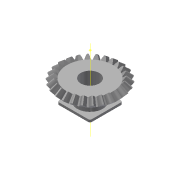
# Autodesk Inventor part: Kegelrad1
Saved by Autodesk Inventor 2017 SP1 (Build 210196100, 196)
## iProperties
Created: 2017-04-24
Part Number: Kegelrad1
Material: Steel, Mild
Document SubType Name: Modeling
Designer: Jochen Alt
Categories: <?xml version="1.0" encoding="UTF-16"?> <MemberInstance><Categories><FamilyTemplate><FamilyTemplateParameter ValueType="xs:double" Id="1" ObjectReferenceKey="da_z" ObjectType="kUserParameterObject"/><FamilyTemplateParameter ValueType="xs:double" Id="2" ObjectReferenceKey="da_b" ObjectType="kUserParameterObject"/><FamilyTemplateParameter ValueType="xs:double" Id="3" ObjectReferenceKey="da_beta" ObjectType="kUserParameterObject"/><FamilyTemplateParameter ValueType="xs:double" Id="4" ObjectReferenceKey="da_dae" ObjectType="kUserParameterObject"/><FamilyTemplateParameter ValueType="xs:double" Id="5" ObjectReferenceKey="da_ve" ObjectType="kUserParameterObject"/><FamilyTemplateParameter ValueType="xs:double" Id="6" ObjectReferenceKey="da_omega" ObjectType="kUserParameterObject"/><FamilyTemplateParameter ValueType="xs:string" Id="7" ObjectReferenceKey="EAIAABAAAAAAHwAAAAAAAIAAAAAAAAAA" ObjectType="83914240" SubObjectId="SurfaceGeometry"/></FamilyTemplate><ParamToTemplateMap><ParamToTemplate CategoryParameter="//CategoryParameter[@InternalName='046C89C9-8512-4d59-83FE-43B91F4F132A']" TemplateParameter="1"/><ParamToTemplate CategoryParameter="//CategoryParameter[@InternalName='2552DF32-E462-4b46-AEBF-C6C7768E72AC']" TemplateParameter="2"/><ParamToTemplate CategoryParameter="//CategoryParameter[@InternalName='C9EE641D-15FC-4fae-A226-E94C4372FDD7']" TemplateParameter="3"/><ParamToTemplate><ParamToTemplate CategoryParameter="//CategoryParameter[@InternalName='00B6519A-459B-49c7-AD84-2E56D39A5744']" ConstantValue="0.000000"/></ParamToTemplate><ParamToTemplate><ParamToTemplate CategoryParameter="//CategoryParameter[@InternalName='04B31F0E-C7A6-4894-AA32-9629BEFACF47']" ConstantValue="1.000000"/></ParamToTemplate><ParamToTemplate><ParamToTemplate CategoryParameter="//CategoryParameter[@InternalName='43CBEC2E-7847-49e7-A936-2F7889FCB2D9']" ConstantValue="0.200000"/></ParamToTemplate><ParamToTemplate><ParamToTemplate CategoryParameter="//CategoryParameter[@InternalName='B1EFC894-105D-4ebd-86BF-FA20ED196853']" ConstantValue="0.266800"/></ParamToTemplate><ParamToTemplate><ParamToTemplate CategoryParameter="//CategoryParameter[@InternalName='51175063-3D10-4879-93E8-6246FE8B403D']" ConstantValue="2060000000.000000"/></ParamToTemplate><ParamToTemplate><ParamToTemplate CategoryParameter="//CategoryParameter[@InternalName='A3A52E27-4454-46a9-B0BD-C932399B70AF']" ConstantValue="0.300000"/></ParamToTemplate><ParamToTemplate CategoryParameter="//CategoryParameter[@InternalName='2A200944-5A8C-41ca-B96E-8520D2E510F1']" TemplateParameter="4"/><ParamToTemplate><ParamToTemplate CategoryParameter="//CategoryParameter[@InternalName='1A637F62-92C8-44bc-B81F-10802510B579']" ConstantValue="2.801056"/></ParamToTemplate><ParamToTemplate CategoryParameter="//CategoryParameter[@InternalName='B52DD4BE-6863-48fb-BF58-89EF6F9EC65C']" TemplateParameter="5"/><ParamToTemplate><ParamToTemplate CategoryParameter="//CategoryParameter[@InternalName='3956BFF2-84D2-457d-93C2-9B0613DEBA67']" ConstantValue="1.153451"/></ParamToTemplate><ParamToTemplate CategoryParameter="//CategoryParameter[@InternalName='739CFA02-461B-4bf8-8049-181FCAD8B28F']" TemplateParameter="6"/><ParamToTemplate><ParamToTemplate CategoryParameter="//CategoryParameter[@InternalName='A27E999F-E2CE-4481-8A2A-EBF499C4C3C5']" ConstantValue="0.000000"/></ParamToTemplate><ParamToTemplate><ParamToTemplate CategoryParameter="//CategoryParameter[@InternalName='9E1B4470-B2D3-4ff1-B813-535BB4CDF51A']" ConstantValue="3520000.000000"/></ParamToTemplate><ParamToTemplate><ParamToTemplate CategoryParameter="//CategoryParameter[@InternalName='F8452263-BFF6-458c-9FB1-07C4B99E95CD']" ConstantValue="11400000.000000"/></ParamToTemplate><ParamToTemplate><ParamToTemplate CategoryParameter="//CategoryParameter[@InternalName='3E3BB259-FD49-497f-8171-6EBC954A3479']" ConstantValue="2.000000"/></ParamToTemplate><ParamToTemplate CategoryParameter="//CategoryParameter[@InternalName='27C3BAF2-7550-4e4b-AE2C-0DB134B7D9B7']" TemplateParameter="7"/></ParamToTemplateMap><Category DisplayName="Gear" InternalName="DC85795E-93AB-48d5-8EEE-5A27447B64BD" Mnemonic="Gear"><CategoryParameter DisplayName="z" InternalName="046C89C9-8512-4d59-83FE-43B91F4F132A" Mnemonic="z"/><CategoryParameter DisplayName="b" InternalName="2552DF32-E462-4b46-AEBF-C6C7768E72AC" Mnemonic="b"/><CategoryParameter DisplayName="||b|" InternalName="C9EE641D-15FC-4fae-A226-E94C4372FDD7" Mnemonic="beta"/><CategoryParameter DisplayName="x" InternalName="00B6519A-459B-49c7-AD84-2E56D39A5744" Mnemonic="x"/><CategoryParameter DisplayName="a*" InternalName="04B31F0E-C7A6-4894-AA32-9629BEFACF47" Mnemonic="a"/><CategoryParameter DisplayName="c*" InternalName="43CBEC2E-7847-49e7-A936-2F7889FCB2D9" Mnemonic="c"/><CategoryParameter DisplayName="r|.f|*" InternalName="B1EFC894-105D-4ebd-86BF-FA20ED196853" Mnemonic="rf"/><CategoryParameter DisplayName="E" InternalName="51175063-3D10-4879-93E8-6246FE8B403D" Mnemonic="E"/><CategoryParameter DisplayName="||m|" InternalName="A3A52E27-4454-46a9-B0BD-C932399B70AF" Mnemonic="mi"/><Category DisplayName="BevelGear" InternalName="0C98F69A-0C2B-4791-B2FE-7691BB227E77" Mnemonic="BevelGear"><CategoryParameter DisplayName="d|.ae|" InternalName="2A200944-5A8C-41ca-B96E-8520D2E510F1" Mnemonic="dae"/><CategoryParameter DisplayName="d|.ai|" InternalName="1A637F62-92C8-44bc-B81F-10802510B579" Mnemonic="dai"/><CategoryParameter DisplayName="A|.e|" InternalName="B52DD4BE-6863-48fb-BF58-89EF6F9EC65C" Mnemonic="ve"/><CategoryParameter DisplayName="A|.i|" InternalName="3956BFF2-84D2-457d-93C2-9B0613DEBA67" Mnemonic="vi"/><CategoryParameter DisplayName="||S|" InternalName="739CFA02-461B-4bf8-8049-181FCAD8B28F" Mnemonic="omega"/><CategoryParameter DisplayName="x|.t|" InternalName="A27E999F-E2CE-4481-8A2A-EBF499C4C3C5" Mnemonic="xt"/><CategoryParameter DisplayName="||s||.Flim|" InternalName="9E1B4470-B2D3-4ff1-B813-535BB4CDF51A" Mnemonic="sFlim"/><CategoryParameter DisplayName="||s||.Hlim|" InternalName="F8452263-BFF6-458c-9FB1-07C4B99E95CD" Mnemonic="sHlim"/><CategoryParameter DisplayName="Typ" InternalName="3E3BB259-FD49-497f-8171-6EBC954A3479" Mnemonic="type"/><CategoryParameter DisplayName="PitchDiameter" InternalName="27C3BAF2-7550-4e4b-AE2C-0DB134B7D9B7" Mnemonic="IDS_PITCHDIAM"/></Category></Category></Categories></MemberInstance>
Mass: 34.6933 g
Surface Area: 30.3012 cm^2
Volume: 4.41953 cm^3
Density: 7.85 g/cm^3
Appearance: Steel
CustomPartVersion: 1
Author: Jochen Alt
Autodesk Inventor part; units mm, degrees
ref_plane "Netzebene2" through (0, 0, 0) normal (0.9927089, 0.1205367, 0) x (0, 0, 1)
sketch "Skizze des Zahnradkörpers" plane through (0, 0, 0) normal (1, 0, 0) x (0, 1, 0)
  line L0 (0, 0) -> (15.2326, -16.1022) construction
  line L1 (15.2326, -16.1022) -> (17.0979, -14.0815)
  line L2 (17.0979, -14.0815) -> (0, 0) construction
  line L3 (16.25, -15) -> (0, 0) construction
  line L4 (12.4774, -13.1897) -> (14.0053, -11.5345)
  line L5 (15.2326, -16.1022) -> (12.4774, -13.1897)
  line L6 (17.0979, -14.0815) -> (14.0053, -11.5345)
  line L7 (0, -19.3226) -> (0, 3.2204) projected
  line L8 (0, -15) -> (17.0979, -15) construction
  dimension "d0" = 32.5
  dimension "d1" = 30.4652
  dimension "d2" = 34.1957
  dimension "d3" = 4
  dimension "d4" = 14.0815
  constraints: 16 end point, 4 point on line, 3 perpendicular, 2 collinear, 1 horizontal alignment, 1 vertical alignment
  measures "d0" diameter of L3.start L7
  measures "d1" diameter of L0.end L7
  measures "d2" diameter of L1.end L7
  measures "d3" distance between parallel lines of L1 L4
  measures "d4" vertical distance of L1.end L0.start
revolve "Zahnradkörper" add sketch "Skizze des Zahnradkörpers" angle 360 about axis through (0, 0, 0) along (0, 0, 1)
ref_plane "Zahnebene" through (0, 16.25, -15) normal (0, -0.7348034, 0.6782801) x (1, 0, 0)
sketch "Startskizze" plane through (0, 16.25, -15) normal (0, -0.7348034, 0.6782801) x (1, 0, 0)
  line L0 (0, -29.1648) -> (0, 7.2852) projected
  arc A0 (-0.2778, -1.83) -> (-2.3077, 1.9725) centre (-10.3357, -4.7562) ccw
  arc A1 (2.3077, 1.9725) -> (0.2778, -1.83) centre (10.3357, -4.7562) ccw
  line L1 (-0.2778, -1.83) -> (0.2778, -1.83)
  arc A2 (2.3077, 1.9725) -> (-2.3077, 1.9725) centre (0, -23.9577) ccw
  dimension "d7" = 10.4749
  dimension "d8" = 10.3357
  dimension "d9" = 19.2015
  dimension "d57" = 26.0327
  dimension "d58" = 22.1276
  constraints: 6 point on circle, 3 centre point, 3 symmetric about line, 2 end point, 1 coincident, 1 perpendicular, 1 other
  measures "d7" radius of A0
  measures "d8" horizontal distance of point (0, -23.958) A0.centre
  measures "d9" vertical distance of point (0, -23.958) A0.centre
  measures "d57" radius of A2
  measures "d58" distance from line of A2.centre L1
ref_plane "Endebene" through (0, 13.2098, -12.1936) normal (0, -0.7348034, 0.6782801) x (1, 0, 0)
sketch "Endskizze" plane through (0, 13.2098, -12.1936) normal (0, -0.7348034, 0.6782801) x (1, 0, 0)
  line L0 (0, -23.7135) -> (0, 5.9534) projected
  arc A0 (-0.2261, -1.4655) -> (-1.8783, 1.6294) centre (-8.4123, -3.8471) ccw
  arc A1 (1.8783, 1.6294) -> (0.2261, -1.4655) centre (8.4123, -3.8471) ccw
  line L1 (-0.2261, -1.4655) -> (0.2261, -1.4655)
  arc A2 (1.8783, 1.6294) -> (-1.8783, 1.6294) centre (0, -19.4754) ccw
  dimension "d12" = 8.5256
  dimension "d15" = 8.4123
  dimension "d16" = 15.6282
  dimension "d59" = 21.1882
  dimension "d60" = 18.0099
  constraints: 6 point on circle, 3 centre point, 3 symmetric about line, 2 end point, 1 coincident, 1 other
  measures "d12" radius of A0
  measures "d15" horizontal distance of A0.centre point (0, -19.475)
  measures "d16" vertical distance of A0.centre point (0, -19.475)
  measures "d59" radius of A2
  measures "d60" distance from line of A2.centre L1
loft "Loft" cut profiles "Startskizze", "Endskizze"
pattern_circular "Circular Pattern" count 26 over 360 about axis through (0, 0, 0) along (0, 0, 1) of "Loft"
sketch3d "3D-Skizze rechts"
ref_plane "Endebene rechts" through (-1.3623, 13.1393, -12.1936) normal (0.0757792, -0.7308855, 0.6782801) x (0.994668, 0.1031285, 0)
sketch "Endskizze rechts" plane through (-1.3623, 13.1393, -12.1936) normal (0.0757792, -0.7308855, 0.6782801) x (0.994668, 0.1031285, 0)
  arc A0 (-0.2261, -1.4655) -> (-1.8783, 1.6294) centre (-8.4123, -3.8471) ccw
  line L0 (0, -25.3523) -> (0, 7.5923) projected
  arc A1 (1.8783, 1.6294) -> (0.2261, -1.4655) centre (8.4123, -3.8471) ccw
  line L1 (-0.2261, -1.4655) -> (0.2261, -1.4655)
  arc A2 (1.8783, 1.6294) -> (-1.8783, 1.6294) centre (0, -19.4754) ccw
  dimension "d70" = 8.4123
  dimension "d71" = 15.6282
  dimension "d72" = 8.5256
  dimension "d73" = 18.0099
  dimension "d74" = 21.1882
  constraints: 6 point on circle, 3 centre point, 3 symmetric about line, 2 end point, 1 coincident, 1 perpendicular, 1 other
  measures "d70" horizontal distance of A2.centre A0.centre
  measures "d71" vertical distance of point (0, -19.475) A0.centre
  measures "d72" radius of A0
  measures "d73" distance from line of point (0, -19.475) L1
  measures "d74" radius of A2
feature "Erhebung rechts" [suppressed]
pattern_circular "Runde Anordnung rechts" [suppressed]
sketch3d "3D-Skizze links"
ref_plane "Endebene links" through (1.3875, 13.1393, -12.206) normal (-0.0771368, -0.7304661, 0.6785788) x (0.9944706, -0.1050155, 0)
sketch "Endskizze links" plane through (1.3875, 13.1393, -12.206) normal (-0.0771368, -0.7304661, 0.6785788) x (0.9944706, -0.1050155, 0)
  line L0 (0, -26.4852) -> (0, 8.7398) projected
  arc A0 (-0.2261, -1.4582) -> (-1.8783, 1.6367) centre (-8.4123, -3.8398) ccw
  arc A1 (1.8783, 1.6367) -> (0.2261, -1.4582) centre (8.4123, -3.8398) ccw
  line L1 (-0.2261, -1.4582) -> (0.2261, -1.4582)
  ellipse E0 centre (0, -8.4724) end of major axis (14.0053, -8.4724) minor radius 9.5037 projected
  arc A2 (1.8783, 1.6367) -> (-1.8783, 1.6367) centre (0, -19.4681) ccw
  dimension "d56" = 9.5037
  dimension "d30" = 8.5256
  dimension "d31" = 8.4123
  dimension "d32" = 15.6282
  dimension "d61" = 21.1882
  dimension "d62" = 18.0099
  constraints: 6 point on circle, 3 centre point, 3 symmetric about line, 2 end point, 1 coincident, 2 other
  measures "d30" radius of A0
  measures "d31" horizontal distance of point (0, -19.468) A0.centre
  measures "d32" vertical distance of A0.centre point (0, -19.468)
  measures "d61" radius of A2
  measures "d62" distance from line of point (0, -19.468) L1
feature "Erhebung links" [suppressed]
pattern_circular "Runde Anordnung links" [suppressed]
sketch "Körperskizze" plane through (0, 0, 0) normal (1, 0, 0) x (0, 1, 0)
  line L0 (0, -16.6847) -> (0, -12.6072) projected
  line L1 (15.2326, -16.1022) -> (12.4774, -13.1897) projected
  line L2 (12.4774, -13.1897) -> (0, -13.1897)
  line L3 (15.2326, -16.1022) -> (0, -16.1022)
  constraints: 4 end point, 2 perpendicular, 2 point on line
revolve "Festkörper" add sketch "Körperskizze" angle 360 about axis through (0, 0, 0) along (0, 0, 1)
sketch "Sketch6" plane through (0, 0, 0) normal (1, 0, 0) x (0, 1, 0)
  line L0 (16.25, -15) -> (0, 0) projected
  line L1 (0, -18) -> (0, 3) projected
surface revolve "Flankendurchmesser" sketch "Sketch6" angle 360 about axis through (0, 0, 0) along (0, 0, 1) shown no curves L0
sketch "Skizze8" plane through (0, 0, -16.1022) normal (0, 0, -1) x (-1, 0, 0)
  arc A0 (3.2767, 14.876) -> (0.3786, 15.2279) centre (0, 0) ccw projected
  circle A1 centre (0, 0) radius 7
  dimension "d94" = 14
  constraints: 1 centre point, 1 coincident
  measures "d94" diameter of A1
ref_plane "Arbeitsebene6" through (-8.9998, -9.0626, -25.4022) normal (0, 0, 1) x (0.9999756, 0.0069813, 0)
extrude "Extrusion1" add sketch "Skizze8" along normal up to surface (9.3 mm away)
chamfer "Fase1" distance 8.2 distance2 6 1 edges at (7, 0, -16.1022) measured on face at (-9.6341, -1.2122, -16.1022)
sketch "Skizze9" plane through (0, 0, -25.4022) normal (0, 0, -1) x (-1, 0, 0)
  circle A0 centre (0, 0) radius 7 projected
  line L0 (7.9, 8.9) -> (-7.9, 8.9)
  line L1 (-8.9, 7.9) -> (-8.9, -7.9)
  line L2 (-7.9, -8.9) -> (7.9, -8.9)
  line L3 (8.9, -7.9) -> (8.9, 7.9)
  line L4 (8.9, 8.9) -> (-8.9, -8.9) construction
  line L5 (-8.9, 8.9) -> (8.9, -8.9) construction
  arc A1 (-8.9, -7.9) -> (-7.9, -8.9) centre (-7.9, -7.9) ccw
  arc A2 (7.9, -8.9) -> (8.9, -7.9) centre (7.9, -7.9) ccw
  arc A3 (8.9, 7.9) -> (7.9, 8.9) centre (7.9, 7.9) ccw
  arc A4 (-7.9, 8.9) -> (-8.9, 7.9) centre (-7.9, 7.9) ccw
  line L6 (-8.9998, 0.0628) -> (-9.0556, -7.937) construction
  arc A5 (-9.0556, -7.937) -> (-8.0626, -8.9439) centre (-8.0557, -7.944) ccw construction
  line L7 (-8.0626, -8.9439) -> (7.937, -9.0556) construction
  arc A6 (7.937, -9.0556) -> (8.9439, -8.0626) centre (7.944, -8.0557) ccw construction
  line L8 (8.9439, -8.0626) -> (8.9998, -0.0628) construction
  line L9 (8.0626, 8.9439) -> (-7.937, 9.0556) construction
  arc A7 (-7.937, 9.0556) -> (-8.9998, 0.0628) centre (-7.944, 8.0557) ccw construction
  line L10 (-8.9439, 8.0626) -> (-8.9998, 0.0628) construction
  arc A8 (8.9998, -0.0628) -> (8.0626, 8.9439) centre (8.0557, 7.944) ccw construction
  line L11 (8.9998, -0.0628) -> (9.0556, 7.937) construction
  dimension "d100" = 17.8
  dimension "d101" = 17.8
  dimension "d102" = 1
  constraints: 12 end point, 8 point on circle, 8 point on line, 8 tangent, 4 centre point, 3 equal radius, 2 midpoint, 2 parallel, 1 horizontal, 1 perpendicular, 2 other
  measures "d100" distance of L5.end L4.end
  measures "d101" distance of L4.end L5.start
  measures "d102" radius of A1
extrude "Extrusion2" add sketch "Skizze9" against normal blind 1.3
sketch "Skizze10" plane through (7.9, -8.9, -25.4022) normal (0, 0, -1) x (-1, 0, 0)
  circle A0 centre (7.9, 8.9) radius 5
  dimension "d105" = 10
  constraints: 1 centre point, 1 coincident
  measures "d105" diameter of A0
extrude "Extrusion3" cut sketch "Skizze10" against normal through all
equation "\"d0\" = da_de"
equation "\"d1\" = da_dfe"
equation "\"d2\" = da_dae"
equation "\"d3\" = da_b"
equation "\"d4\" = da_ve"
equation "\"d7\" = fd_rr"
equation "\"d8\" = fd_x"
equation "\"d9\" = fd_y"
equation "\"d57\" = 0.5 * fd_dva + 0.3 * da_he"
equation "\"d58\" = 0.5 * fd_dva - 1.12 * da_he"
equation "\"da_teethtype\" = 0"
equation "\"da_b\" = 4"
equation "\"da_de\" = 32.5"
equation "\"da_dae\" = 34.1957"
equation "\"da_dfe\" = 30.46516"
equation "\"da_le\" = 22.11476"
equation "\"da_omega\" = 90deg"
equation "\"da_beta\" = 0"
equation "\"da_delta\" = 47.29061deg"
equation "\"da_alpha\" = 25deg"
equation "\"da_he\" = 2.75"
equation "\"da_ve\" = 14.0815"
equation "\"da_zv\" = 38.332246"
equation "\"fd_loft\" = da_b + 0.05 * da_he"
equation "\"fd_x\" = fd_x1 + fd_x2"
equation "\"fd_y\" = fd_y1 - fd_y2"
equation "\"fd_dd\" = fd_dva - 0.8 * da_he"
equation "\"da_dvw\" = 47.91531"
equation "\"d11\" = fd_loft"
equation "\"da_dm\" = 29.56079"
equation "\"da_x\" = 0"
equation "\"da_m\" = 1.25"
equation "\"d50\" = da_omega"
equation "\"fd_rr\" = 10.474934"
equation "\"fd_dva\" = 50.415308"
equation "\"fd_x1\" = 0.992372"
equation "\"fd_x2\" = 9.343349"
equation "\"fd_y1\" = 23.937092"
equation "\"fd_y2\" = 4.735617"
body "Solid1"
body "Srf1"
